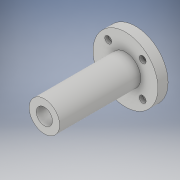
# Autodesk Inventor part: LMF8LUU
Saved by Autodesk Inventor 2018 (Build 220112000, 112)
## iProperties
Created: 2017-10-09
Part Number: LMF8LUU
Material: Generic
Document SubType Name: Modeling
Designer: Jurjen
Density: 1 g/cm^3
Appearance: Default
Author: Jurjen
Autodesk Inventor part; units mm, degrees
ref_plane "YZ Plane" through (0, 0, 0) normal (1, 0, 0) x (0, 1, 0)
ref_plane "XZ Plane" through (0, 0, 0) normal (0, 1, 0) x (-1, 0, 0)
ref_plane "XY Plane" through (0, 0, 0) normal (0, 0, 1) x (1, 0, 0)
sketch "Sketch1" plane through (0, 0, 0) normal (0, 1, 0) x (-1, 0, 0)
  line L0 (0, 22.5) -> (7.5, 22.5)
  line L1 (7.5, 22.5) -> (7.5, -17.5)
  line L2 (7.5, -17.5) -> (16, -17.5)
  line L3 (16, -17.5) -> (16, -22.5)
  line L4 (16, -22.5) -> (0, -22.5)
  line L5 (0, -22.5) -> (0, 22.5)
  point P0 (0, 0)
  point P1 (0, 0)
  dimension "d0" = 7.5
  dimension "d1" = 5
  dimension "d3" = 16
  dimension "d4" = 45
  constraints: 12 end point, 5 perpendicular, 1 coincident, 1 horizontal, 1 midpoint, 1 vertical alignment
  measures "d0" distance between parallel lines of L1 L5
  measures "d1" distance of L2.end L3.end
  measures "d3" distance of L3.end L4.end
  measures "d4" distance between parallel lines of L4 L0
revolve "Revolution1" add sketch "Sketch1" angle 360 about axis through (0, 0, -22.5) along (0, 0, 1)
sketch "Sketch2" plane through (0, 0, 22.5) normal (0, 0, 1) x (1, 0, 0)
  circle A0 centre (0, 0) radius 4
  dimension "d5" = 8
  constraints: 1 centre point, 1 coincident
  measures "d5" diameter of A0
extrude "Extrusion1" cut sketch "Sketch2" against normal up to next
sketch "Sketch3" plane through (0, 0, -17.5) normal (0, 0, 1) x (1, 0, 0)
  circle A0 centre (-8.4853, 8.4853) radius 1.7
  line L0 (0, 0) -> (-8.4853, 8.4853) construction
  line L1 (0, 0) -> (-3.1591, 0)
  circle A1 centre (-8.4853, -8.4853) radius 1.7
  circle A2 centre (8.4853, -8.4853) radius 1.7
  circle A3 centre (8.4853, 8.4853) radius 1.7
  dimension "d8" = 3.4
  dimension "d9" = 12
  dimension "d10" = 45
  dimension "d13" = 360
  constraints: 4 centre point, 4 end point, 1 horizontal, 9 other
  measures "d8" diameter of A0
  measures "d9" distance of L0.start L0.end
  measures "d10" angle of L0 L1
extrude "Extrusion2" cut sketch "Sketch3" against normal up to next
sketch "Sketch4" plane through (0, 0, -22.5) normal (0, 0, -1) x (-1, 0, 0)
  circle A0 centre (8.4853, 8.4853) radius 1.7 projected
  circle A1 centre (8.4853, 8.4853) radius 3.25
  circle A2 centre (-8.4853, 8.4853) radius 3.25
  circle A3 centre (-8.4853, -8.4853) radius 3.25
  circle A4 centre (8.4853, -8.4853) radius 3.25
  point P0 (0, 0)
  dimension "d17" = 6.5
  dimension "d20" = 360
  constraints: 4 centre point, 1 coincident, 9 other
  measures "d17" diameter of A1
extrude "Extrusion3" cut sketch "Sketch4" against normal blind 3.3
body "Solid1"
